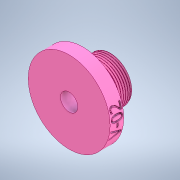
# Autodesk Inventor part: brakeHandle
Saved by Autodesk Inventor 2021.1 (Build 251245000, 245)
## iProperties
Created: 2020-08-18
Part Number: brakeHandle
Material: Polycarbonate, Smoke
Document SubType Name: Modeling
Designer: robst
Density: 1.2 g/cm^3
Appearance: Pink
innerDiameter: 0.635 in
heightOfBrake: 0.250 in
majorDiameter: 1.623 in
pitchDiameter: 1.569 in
minorDiameter: 1.524 in
pitch: 0.083 in
crestFlat: 0.017 in
rootRadius: 0.009 in
threadsPerInch: 12.000 ul
threadDepth: 0.060 in
Author: robst
Autodesk Inventor part; units mm, degrees
ref_plane "XZ Plane" through (0, 0, 0) normal (0, 1, 0) x (-1, 0, 0)
ref_plane "XY Plane" through (0, 0, 0) normal (0, 0, 1) x (1, 0, 0)
sketch "Sketch1" plane through (0, 0, 0) normal (0, 0, 1) x (1, 0, 0)
  circle A0 centre (0, 0) radius 8.0645
  circle A1 centre (0, 0) radius 20.5061
  dimension "d0" = 16.129
  dimension "d1" = 41.0121
  constraints: 2 centre point, 2 coincident
  measures "d0" diameter of A0
  measures "d1" diameter of A1
extrude "Extrusion1" add sketch "Sketch1" against normal blind 25.4
sketch "Sketch2" plane through (0, 0, 0) normal (0, 0, 1) x (1, 0, 0)
  circle A0 centre (0, 0) radius 8.0645
  circle A1 centre (0, 0) radius 38.1
  dimension "d4" = 76.2
  dimension "d56" = 16.129
  constraints: 2 centre point, 2 coincident
  measures "d4" diameter of A1
  measures "d56" diameter of A0
extrude "Extrusion2" add sketch "Sketch2" along normal blind 12.7
sketch "Sketch9" plane through (0, 0, 0) normal (1, 0, 0) x (0, 1, 0)
  line L0 (20.5061, 0) -> (20.5061, -25.4) projected
  line L1 (-20.5061, -25.4) -> (20.5061, -25.4) projected
  line L2 (20.5061, -27.5167) -> (19.3002, -28.2129)
  line L3 (19.3002, -28.6) -> (20.5061, -29.2962)
  arc A0 (19.3002, -28.2129) -> (19.3002, -28.6) centre (19.412, -28.4064) ccw
  line L4 (20.5061, -27.5167) -> (20.5061, -29.2962)
  line L5 (0, -25.4) -> (0, -43.7839) construction
  point P0 (0, 0)
  dimension "d38" = 60
  dimension "d39" = 0.2235
  dimension "d41" = 2.1167
  dimension "d42" = 20.506
  dimension "d52" = 19.1884
  constraints: 8 end point, 2 point on circle, 2 tangent, 2 vertical, 1 centre point, 1 equal length, 1 midpoint
  measures "d38" angle of L3 L2
  measures "d39" radius of A0
  measures "d41" distance from line of L2.start L1
  measures "d42" distance from line of L4 point (0, 0)
  measures "d52" distance edge to line of A0 L5
coil "Coil2" sketch "Sketch9" operation cut axis through (0, 0, -10) along (0, 0, 1) pitch 2.1167 turns 14 hand right
ref_plane "Work Plane1" through (38.1, 0, 0) normal (1, 0, 0) x (0, 1, 0)
sketch "Sketch10" plane through (38.1, 0, 0) normal (1, 0, 0) x (0, 1, 0)
  line L0 (38.1, 0) -> (38.1, 12.7) construction
  line L1 (38.1, 6.35) -> (-38.1, 6.35) construction
  line L2 (-38.1, 0) -> (-38.1, 12.7) construction
  line L3 (-5.9322, 11.43) -> (-9.4313, 1.27)
  line L4 (-9.4313, 1.27) -> (-10.8887, 1.27)
  line L5 (-10.8887, 1.27) -> (-14.3878, 11.43)
  line L6 (-14.3878, 11.43) -> (-12.9388, 11.43)
  line L7 (-12.9388, 11.43) -> (-10.1229, 2.9908)
  line L8 (-10.1229, 2.9908) -> (-7.3071, 11.43)
  line L9 (-7.3071, 11.43) -> (-5.9322, 11.43)
  line L10 (-1.412, 5.0985) -> (-5.257, 5.0985)
  line L11 (-5.257, 5.0985) -> (-5.257, 6.3335)
  line L12 (-5.257, 6.3335) -> (-1.412, 6.3335)
  line L13 (-1.412, 6.3335) -> (-1.412, 5.0985)
  spline S0 degree 2 poles (6.2615, 6.35) (6.2615, 3.6165) (4.6724, 1.0559) (3.0175, 1.0559) knots 0 0 0 1 2 2 2
  spline S1 degree 2 poles (3.0175, 1.0559) (1.3379, 1.0559) (-0.2347, 3.6659) (-0.2347, 6.3418) knots 0 0 0 1 2 2 2
  spline S2 degree 2 poles (-0.2347, 6.3418) (-0.2347, 9.0917) (1.3544, 11.6358) (3.0175, 11.6358) knots 0 0 0 1 2 2 2
  spline S3 degree 2 poles (3.0175, 11.6358) (4.6889, 11.6358) (6.2615, 9.0012) (6.2615, 6.35) knots 0 0 0 1 2 2 2
  spline S4 degree 2 poles (4.516, 3.2542) (4.7136, 3.7565) (4.8783, 5.3044) (4.8783, 6.35) knots 0 0 0 1 2 2 2
  spline S5 degree 2 poles (4.8783, 6.35) (4.8783, 7.3956) (4.7136, 8.9353) (4.5078, 9.454) knots 0 0 0 1 2 2 2
  spline S6 degree 2 poles (4.5078, 9.454) (4.3019, 9.9727) (3.5856, 10.5079) (3.0175, 10.5079) knots 0 0 0 1 2 2 2
  spline S7 degree 2 poles (3.0175, 10.5079) (2.4494, 10.5079) (1.7167, 9.9727) (1.5026, 9.4375) knots 0 0 0 1 2 2 2
  spline S8 degree 2 poles (1.5026, 9.4375) (1.2968, 8.9188) (1.1486, 7.338) (1.1486, 6.3418) knots 0 0 0 1 2 2 2
  spline S9 degree 2 poles (1.1486, 6.3418) (1.1486, 5.2714) (1.2803, 3.8388) (1.4944, 3.2789) knots 0 0 0 1 2 2 2
  spline S10 degree 2 poles (1.4944, 3.2789) (1.692, 2.752) (2.4247, 2.1839) (3.0175, 2.1839) knots 0 0 0 1 2 2 2
  spline S11 degree 2 poles (3.0175, 2.1839) (3.5774, 2.1839) (4.3102, 2.7191) (4.516, 3.2542) knots 0 0 0 1 2 2 2
  line L14 (13.828, 1.27) -> (7.5624, 1.27)
  line L15 (7.5624, 1.27) -> (7.5624, 2.7108)
  spline S12 degree 2 poles (7.5624, 2.7108) (8.2375, 3.3448) (9.4396, 4.5222) (10.0159, 5.1562) knots 0 0 0 1 2 2 2
  spline S13 degree 2 poles (10.0159, 5.1562) (11.1768, 6.4323) (12.0249, 7.9637) (12.0249, 8.7788) knots 0 0 0 1 2 2 2
  spline S14 degree 2 poles (12.0249, 8.7788) (12.0249, 9.207) (11.7614, 9.8492) (11.5226, 10.055) knots 0 0 0 1 2 2 2
  spline S15 degree 2 poles (11.5226, 10.055) (11.2839, 10.2609) (10.6581, 10.4667) (10.2794, 10.4667) knots 0 0 0 1 2 2 2
  spline S16 degree 2 poles (10.2794, 10.4667) (9.9171, 10.4667) (9.1761, 10.2856) (8.8385, 10.1456) knots 0 0 0 1 2 2 2
  spline S17 degree 2 poles (8.8385, 10.1456) (8.5504, 10.0303) (8.0152, 9.701) (7.8505, 9.5857) knots 0 0 0 1 2 2 2
  line L16 (7.8505, 9.5857) -> (7.7764, 9.5857)
  line L17 (7.7764, 9.5857) -> (7.7764, 11.0348)
  spline S18 degree 2 poles (7.7764, 11.0348) (8.1963, 11.2406) (9.703, 11.6441) (10.3782, 11.6441) knots 0 0 0 1 2 2 2
  spline S19 degree 2 poles (10.3782, 11.6441) (11.8026, 11.6441) (13.4081, 10.1374) (13.4081, 8.8529) knots 0 0 0 1 2 2 2
  spline S20 degree 2 poles (13.4081, 8.8529) (13.4081, 8.2519) (13.1281, 7.2474) (12.8811, 6.8193) knots 0 0 0 1 2 2 2
  spline S21 degree 2 poles (12.8811, 6.8193) (12.6341, 6.3747) (11.9178, 5.502) (11.5226, 5.0821) knots 0 0 0 1 2 2 2
  spline S22 degree 2 poles (11.5226, 5.0821) (10.8804, 4.3822) (9.3078, 2.8837) (8.8385, 2.4474) knots 0 0 0 1 2 2 2
  line L18 (8.8385, 2.4474) -> (13.828, 2.4474)
  line L19 (13.828, 2.4474) -> (13.828, 1.27)
  point P0 (0, 0)
  constraints: 2 end point, 2 midpoint, 1 horizontal
emboss "Emboss1" sketch "Sketch10" operation cut depth 2.54 direction (-1, 0, 0) wrap yes faces at (37.6745, -5.6785, 8.4667)
equation "\"d0\" = innerDiameter"
equation "\"d1\" = a1MajorDiameterAvg"
equation "\"d2\" = threadPostLength"
equation "\"d4\" = handleDiameter"
equation "\"d56\" = innerDiameter"
equation "\"d5\" = handleLength"
equation "\"d39\" = rootRadius"
equation "\"d41\" = pitch"
equation "\"d42\" = 0.5 * a1MajorDiameterAvg"
equation "\"d52\" = 0.5 * a1MinorDiameterAvg"
equation "\"d43\" = pitch"
equation "\"d44\" = threadLength"
equation "\"handleDiameter\" = 76.2"
equation "\"brakeHandle\" = 30deg"
equation "\"innerDiameter\" = 16.129"
equation "\"heightOfBrake\" = 6.35"
equation "\"majorDiameter\" = 41.22928"
equation "\"pitchDiameter\" = 39.85514"
equation "\"minorDiameter\" = 38.7096"
equation "\"crestFlat\" = 0.4318"
equation "\"rootRadius\" = 0.22352"
equation "\"threadsPerInch\" = 12"
equation "\"threadDepth\" = 1.52146"
equation "\"d53\" = 0.5 * handleDiameter"
equation "\"totalLength\" = 38.1"
equation "\"handleLength\" = 12.7"
equation "\"threadPostLength\" = totalLength - handleLength"
equation "\"threadLength\" = threadPostLength + 2 * pitch"
equation "\"brakeStopLength\" = 12.7"
equation "\"a1MajorDiameterMax\" = 41.22928"
equation "\"a1MajorDiameterMin\" = 40.79494"
equation "\"a1MajorDiameterAvg\" = 0.5 * a1MajorDiameterMin + 0.5 * a1MajorDiameterMax"
equation "\"a1MinorDiameterMax\" = 38.7096"
equation "\"a1MinorDiameterMin\" = 38.04412"
equation "\"a1MinorDiameterAvg\" = 0.5 * a1MinorDiameterMin + 0.5 * a1MinorDiameterMax"
equation "\"a1RootRadiusMax\" = 0.26162"
equation "\"a1RootRadiusMin\" = 0.1524"
equation "\"a1RootRadiusAvg\" = 0.5 * a1RootRadiusMin + 0.5 * a1RootRadiusMax"
equation "\"pitch\" = 2.116667"
body "Solid1"
